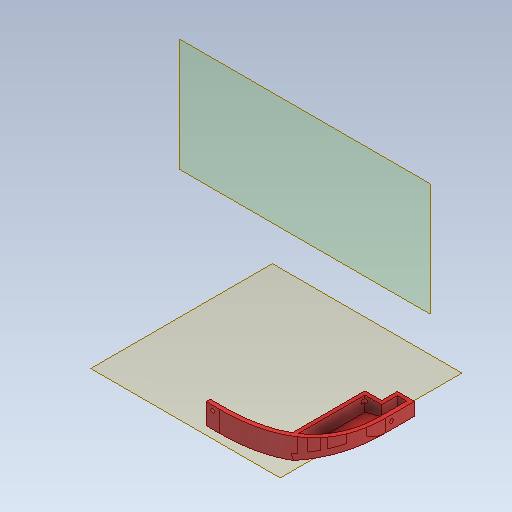
# Autodesk Inventor part: canto
Saved by Autodesk Inventor 2020 (Build 240168000, 168)
## iProperties
Created: 2020-04-24
Part Number: canto
Material: Genérico
Document SubType Name: Modeling
Designer: gi-se
Density: 1 g/cm^3
Appearance: Vermelho alaranjado
Author: gi-se
Autodesk Inventor part; units mm, degrees
ref_plane "YZ Plane" through (0, 0, 0) normal (1, 0, 0) x (0, 1, 0)
ref_plane "XZ Plane" through (0, 0, 0) normal (0, 1, 0) x (-1, 0, 0)
ref_plane "XY Plane" through (0, 0, 0) normal (0, 0, 1) x (1, 0, 0)
ref_plane "Plano de trabalho1" through (4.85, -66.1, 3.317814) normal (0, 1, 0) x (-1, 0, 0)
sketch "Esboço7" plane through (4.85, -66.1, 3.317814) normal (0, 1, 0) x (-1, 0, 0)
  spline S0 degree 4 poles (-63.15, 3.682186) (-63.142335, 9.732075) (-62.18363, 17.577122) (-58.839618, 26.416885) (-51.359365, 34.601206) (-41.420425, 41.161438) (-30.747731, 43.972695) (-21.220771, 44.813565) (-13.75, 44.817814) knots 0 0 0 0 0 0.30669719 0.4235016 0.54102531 0.66311948 1 1 1 1 1
  line L0 (0.45, -30.926645) -> (0.45, -16.417814)
  line L1 (14.341169, -44.817814) -> (0.45, -30.926645)
  line L2 (46.75, -44.817814) -> (14.341169, -44.817814)
  line L3 (46.75, 25.38432) -> (46.75, -44.817814)
  line L4 (-9.75, 35.346795) -> (46.75, 25.38432)
  line L5 (-6.75, 44.817814) -> (-6.75, 38.346795)
  line L6 (-13.75, 44.817814) -> (-6.75, 44.817814)
  spline S1 degree 2 poles (-46.75, 37.469642) (-34.671162, 44.817814) (-13.75, 44.817814) knots 0 0 0 1 1 1
  line L7 (-46.75, -44.817814) -> (-46.75, 37.469642)
  line L8 (4.158831, -44.817814) -> (-46.75, -44.817814)
  line L9 (-5.695584, -34.963398) -> (4.158831, -44.817814)
  arc A0 (-6.75, -32.417814) -> (-5.695584, -34.963398) centre (-3.15, -32.417814) ccw
  line L10 (-6.75, -16.417814) -> (-6.75, -32.417814)
  arc A1 (0.45, -16.417814) -> (-6.75, -16.417814) centre (-3.15, -16.417814) ccw
  circle A2 centre (-14.05, -11.017814) radius 0.8
  line L11 (-63.15, 3.682186) -> (-44.75, 3.682186)
  line L12 (-6.75, 42.567814) -> (-6.75, 44.817814)
  line L13 (-6.75, 44.817814) -> (-13.75, 44.817814)
  line L14 (-60.858893, 5.932186) -> (-44.75, 5.932186)
  line L15 (-9, 42.567814) -> (-13.75, 42.567814)
  line L16 (-44.75, 41.3031) -> (-44.75, 2)
  line L17 (-9, 42.567814) -> (-6.75, 42.567814)
  line L18 (-6.75, 44.817814) -> (-6.75, 42.567814)
  line L19 (-6.75, 42.567814) -> (-9.75, 42.567814)
  line L20 (-9.75, 42.567814) -> (-9.75, 44.817814)
  line L21 (-9.75, 44.817814) -> (-6.75, 44.817814)
  line L22 (-9.75, 38.346795) -> (-9.75, 35.346795)
  line L23 (-6.75, 38.346795) -> (-9.75, 38.346795)
  spline S2 degree 5 poles (-13.748721, 42.567814) (-17.011521, 42.565862) (-20.274495, 42.452633) (-23.531674, 42.205009) (-29.595553, 41.442064) (-35.526192, 39.976484) (-38.23954, 39.119482) (-43.237503, 37.094016) (-47.789537, 34.213647) (-49.802218, 32.646807) (-53.452771, 29.089024) (-56.245096, 24.82436) (-57.399397, 22.545019) (-59.2024, 17.936427) (-60.232691, 13.096486) (-60.5712, 10.718215) (-60.773011, 8.327267) (-60.858895, 5.932186) knots 0 0 0 0 0 0 0.24056469 0.24056469 0.24056469 0.44973286 0.44973286 0.44973286 0.6363542 0.6363542 0.6363542 0.82330304 0.82330304 0.82330304 1 1 1 1 1 1
  point P0 (4.85, -3.317814)
  point P1 (-62.348789, 13.492523)
  point P2 (-60.046821, 21.718124)
  point P3 (-56.342657, 28.55399)
  point P4 (-51.235855, 34.164448)
  point P5 (-44.620354, 38.639423)
  point P6 (-36.311689, 41.974216)
  point P7 (-26.092384, 44.080443)
  point P8 (-46.75, 5.932186)
  point P9 (-46.75, 34.756638)
  point P10 (-44.75, 35.999842)
  point P11 (-13.749358, 42.567814)
  point P12 (-46.75, 3.682186)
  dimension "d24" = 2
  dimension "d37" = 3
  constraints: 22 end point, 6 perpendicular, 4 parallel, 2 point on line, 13 other
  measures "d24" distance between parallel lines of L7 L16
  measures "d37" distance of L12.start L19.end
sketch "Esboço7 outline for Extrusão6" plane through (4.85, -66.1, 3.317814) normal (0, 1, 0) x (-1, 0, 0)
  line L0 (-44.75, 3.682186) -> (-44.750011, 35.999861)
  spline S0 degree 5 poles (-13.748721, 42.567814) (-17.011521, 42.565862) (-20.274495, 42.452633) (-23.531674, 42.205009) (-29.595553, 41.442064) (-35.526192, 39.976484) (-38.23954, 39.119482) (-41.167958, 37.932717) (-43.943286, 36.452458) (-44.213822, 36.304492) (-44.482758, 36.153642) (-44.750023, 35.999881) knots 0 0 0 0 0 0 0.50916763 0.50916763 0.50916763 0.95188291 0.95188291 0.95188291 1 1 1 1 1 1
  line L1 (-13.748721, 42.567814) -> (-9.75, 42.567814)
  line L2 (-9.75, 42.567814) -> (-9.75, 44.817814)
  line L3 (-9.75, 44.817814) -> (-13.75, 44.817814)
  spline S1 degree 4 poles (-63.15, 3.682186) (-63.142335, 9.732075) (-62.18363, 17.577122) (-58.839618, 26.416885) (-51.359365, 34.601206) (-41.420425, 41.161438) (-30.747731, 43.972695) (-21.220771, 44.813565) (-13.75, 44.817814) knots 0 0 0 0 0 0.30669719 0.4235016 0.54102531 0.66311948 1 1 1 1 1
  line L4 (-63.15, 3.682186) -> (-44.75, 3.682186)
  line L5 (-46.75, 5.932186) -> (-60.858895, 5.932186)
  spline S2 degree 5 poles (-46.749999, 34.756636) (-48.204588, 33.780364) (-49.594289, 32.707372) (-50.905012, 31.535519) (-53.882304, 28.433006) (-56.245096, 24.82436) (-57.399397, 22.545019) (-59.2024, 17.936427) (-60.232691, 13.096486) (-60.5712, 10.718215) (-60.773011, 8.327267) (-60.858895, 5.932186) knots 0 0 0 0 0 0 0.26208571 0.26208571 0.26208571 0.64144447 0.64144447 0.64144447 1 1 1 1 1 1
  line L6 (-46.75, 34.756638) -> (-46.75, 5.932186)
extrude "Extrusão6" add sketch "Esboço7 outline for Extrusão6" along normal blind 11.3
sketch "Esboço8" plane through (68, -66.1, 7) normal (0, 0, -1) x (-1, 0, 0)
  line L0 (16.4, 0) -> (16.4, 11.3) projected
  line L1 (16.4, 0) -> (0, 4.3)
  line L2 (0, 4.3) -> (-5, 0)
  line L3 (-5, 0) -> (12, -6)
  line L4 (12, -6) -> (16.4, 0)
  point P0 (68, 66.1)
  constraints: 8 end point, 1 other
sketch "Esboço8 outline for Extrusão7" plane through (68, -66.1, 7) normal (0, 0, -1) x (-1, 0, 0)
  line L0 (0, 4.3) -> (-5, 0)
  line L1 (16.4, 0) -> (0, 4.3)
  line L2 (12, -6) -> (16.4, 0)
  line L3 (-5, 0) -> (12, -6)
extrude "Extrusão7" cut sketch "Esboço8 outline for Extrusão7" against normal blind 48.25
sketch "Esboço9" plane through (68, -54.8, 7) normal (0, 0, -1) x (-1, 0, 0)
  line L0 (16.4, -11.3) -> (2.291107, -7.600717)
  line L1 (0, -7) -> (0, 0)
  line L2 (16.4, -11.3) -> (0, -7)
  line L3 (0, -7) -> (0.800313, -3.947643)
  line L4 (0.800313, -3.947643) -> (17.200313, -8.247643)
  line L5 (17.200313, -8.247643) -> (16.4, -11.3)
  point P0 (68, 54.8)
  constraints: 8 end point, 2 parallel, 1 perpendicular
sketch "Esboço9 outline for Extrusão8" plane through (68, -54.8, 7) normal (0, 0, -1) x (-1, 0, 0)
  line L0 (16.4, -11.3) -> (17.200313, -8.247643)
  line L1 (2.291107, -7.600717) -> (16.4, -11.3)
  line L2 (0, -7) -> (2.291107, -7.600717)
  line L3 (0.800313, -3.947643) -> (0, -7)
  line L4 (17.200313, -8.247643) -> (0.800313, -3.947643)
extrude "Extrusão8" add sketch "Esboço9 outline for Extrusão8" against normal blind 48
sketch "Esboço10" plane through (4.85, -54.8, 3.317814) normal (0, 1, 0) x (1, 0, 0)
  spline S0 degree 2 poles (63.15, -3.682186) (63.15, -44.817814) (13.75, -44.817814) knots 1 1 1 2 2 2
  line L0 (63.15, -3.682186) -> (46.75, -3.682186)
  line L1 (63.15, -3.682186) -> (63.15, -51.682186)
  line L2 (63.15, -51.682186) -> (45.949687, -51.682186)
  line L3 (45.949687, -51.682186) -> (45.949687, -3.682186)
  line L4 (45.949687, -3.682186) -> (63.15, -3.682186)
  point P0 (-4.85, 3.317814)
  point P1 (45.949687, -37.905329)
  constraints: 8 end point, 2 parallel, 1 perpendicular, 1 vertical
sketch "Esboço10 outline for Extrusão9" plane through (4.85, -54.8, 3.317814) normal (0, 1, 0) x (1, 0, 0)
  line L0 (45.949687, -51.682186) -> (63.15, -51.682186)
  line L1 (45.949687, -37.905329) -> (45.949687, -51.682186)
  spline S0 degree 2 poles (63.15, -3.682186) (63.15, -27.955151) (45.949687, -37.905329) knots 0 0 0 1 1 1
  line L2 (63.15, -51.682186) -> (63.15, -3.682186)
extrude "Extrusão9" cut sketch "Esboço10 outline for Extrusão9" against normal blind 48
sketch "Esboço11" plane through (68, -54.8, 7) normal (0, 0, -1) x (-1, 0, 0)
  line L0 (16.4, -11.3) -> (18.4, -11.3) projected
  line L1 (18.4, -11.3) -> (18.4, 0) projected
  line L2 (0, 0) -> (18.4, 0) projected
  line L3 (0, -7) -> (0, 0) projected
  line L4 (0, -7) -> (16.4, -11.3) projected
  line L5 (16.4, -11.3) -> (0, 14.8) projected
  point P0 (68, 54.8)
  point P1 (9.299617, 0)
sketch "Esboço11 outline for Extrusão10" plane through (68, -54.8, 7) normal (0, 0, -1) x (-1, 0, 0)
  line L0 (0, 0) -> (0, -7)
  line L1 (9.299617, 0) -> (0, 0)
  line L2 (16.4, -11.3) -> (9.299617, 0)
  line L3 (0, -7) -> (16.4, -11.3)
extrude "Extrusão10" add sketch "Esboço11 outline for Extrusão10" along normal blind 15.5
sketch "Esboço12" plane through (49.6, -66.1, 7) normal (0, 0, -1) x (-1, 0, 0)
  line L0 (91.5, 0) -> (-2, 0)
  line L1 (117.6, 26.1) -> (91.5, 0)
  line L2 (117.6, 50.1) -> (117.6, 26.1)
  line L3 (93.6, 50.1) -> (117.6, 50.1)
  line L4 (93.6, 82.1) -> (93.6, 50.1)
  line L5 (117.6, 82.1) -> (93.6, 82.1)
  line L6 (117.6, 106.1) -> (117.6, 82.1)
  line L7 (91.5, 132.2) -> (117.6, 106.1)
  line L8 (-2, 132.2) -> (91.5, 132.2)
  line L9 (-18.4, 106.1) -> (-2, 132.2)
  line L10 (-18.4, 26.1) -> (-18.4, 106.1)
  line L11 (-2, 0) -> (-18.4, 26.1)
  spline S0 degree 3 poles (-7.815486, 104.038144) (-7.816082, 104.037708) (-7.816681, 104.03727) (-7.846099, 104.015744) (-7.882015, 103.988404) (-7.95841, 103.925869) (-7.998834, 103.890604) (-8.072489, 103.822008) (-8.110537, 103.784191) (-8.178341, 103.712432) (-8.208164, 103.678549) (-8.253706, 103.624789) (-8.272728, 103.601104) (-8.285509, 103.584876) knots 0 0 0 0 0.00416713 0.00416713 0.20441217 0.20441217 0.40465722 0.40465722 0.60490226 0.60490226 0.8051473 0.8051473 1 1 1 1
  arc A0 (-8.285509, 103.584876) -> (-7.815486, 104.038144) centre (-6.4, 102.1) ccw
  spline S1 degree 3 poles (-7.84364, 32.017255) (-7.866833, 31.999781) (-7.892941, 31.97946) (-7.95841, 31.925869) (-7.998834, 31.890604) (-8.072489, 31.822008) (-8.110537, 31.784191) (-8.168644, 31.722696) (-8.190769, 31.698097) (-8.209846, 31.676205) knots 0 0 0 0 0.20827667 0.20827667 0.5 0.5 0.79172333 0.79172333 1 1 1 1
  arc A1 (-8.209846, 31.676205) -> (-7.84364, 32.017255) centre (-6.4, 30.1) ccw
  line L12 (-2, 11.3) -> (-16.108893, 11.3)
  line L13 (-9.054446, 11.3) -> (0, 11.3)
  line L14 (0, 11.3) -> (0, 0)
  point P0 (49.6, 66.1)
  point P1 (-9.100383, 11.3)
  constraints: 4 end point, 1 horizontal, 1 midpoint, 1 perpendicular, 1 point on line
sketch "Esboço12 outline for Extrusão11" plane through (49.6, -66.1, 7) normal (0, 0, -1) x (-1, 0, 0)
  line L0 (0, 0) -> (0, 11.3)
  line L1 (-2, 0) -> (0, 0)
  line L2 (-9.100383, 11.3) -> (-2, 0)
  line L3 (-2, 11.3) -> (-9.100383, 11.3)
  line L4 (0, 11.3) -> (-2, 11.3)
extrude "Extrusão11" add sketch "Esboço12 outline for Extrusão11" along normal blind 7
sketch "Esboço13" plane through (4.85, -54.8, 3.317814) normal (0, 1, 0) x (1, 0, 0)
  line L0 (46.75, -34.756638) -> (46.75, -5.932186)
  line L1 (46.75, -5.932186) -> (60.858893, -5.932186)
  line L2 (60.858893, -5.932186) -> (60.858893, 1.317814)
  line L3 (55.850383, 1.317814) -> (46.75, 1.317814)
  line L4 (46.75, 1.317814) -> (46.75, -5.932186)
  line L5 (63.15, -3.682186) -> (63.15, 11.817814)
  line L6 (44.75, 3.317814) -> (53.850383, 3.317814)
  line L7 (60.858893, 1.305176) -> (60.858893, 9.817814)
  line L8 (60.858893, 9.817814) -> (55.850383, 9.817814)
  line L9 (55.850383, 9.817814) -> (55.850383, 1.317814)
  line L10 (53.850383, 3.317814) -> (53.850383, 11.817814)
  line L11 (53.850383, 11.817814) -> (63.15, 11.817814)
  line L12 (63.15, -3.682186) -> (63.15, 11.817814)
  line L13 (53.850383, 11.817814) -> (63.15, 11.817814)
  line L14 (53.850383, 3.317814) -> (53.850383, 11.817814)
  line L15 (44.75, 3.317814) -> (53.850383, 3.317814)
  line L16 (44.75, -35.999842) -> (44.75, 3.317814)
  line L17 (13.748721, -42.567814) -> (9.75, -42.567814)
  line L18 (9.75, -42.567814) -> (9.75, -44.817814)
  line L19 (9.75, -44.817814) -> (13.75, -44.817814)
  line L20 (46.75, -5.932186) -> (60.858893, -5.932186)
  line L21 (46.75, -34.756638) -> (46.75, -5.932186)
  point P0 (-4.85, 3.317814)
  point P1 (60.858893, 1.317814)
  dimension "d39" = 2
  dimension "d40" = 2
  dimension "d41" = 2
  dimension "d42" = 0
  dimension "d43" = 0
  constraints: 14 end point, 3 parallel, 1 horizontal, 1 perpendicular, 9 other
  measures "d39" distance between parallel lines of L3 L6
  measures "d40" distance between parallel lines of L10 L9
  measures "d41" distance between parallel lines of L8 L11
  measures "d42" distance from line of L20.end L2
  measures "d43" distance between parallel lines of L7 L2
sketch "Esboço13 outline for Extrusão12" plane through (4.85, -54.8, 3.317814) normal (0, 1, 0) x (1, 0, 0)
  line L0 (46.75, 1.317814) -> (46.75, -5.932186)
  line L1 (55.850383, 1.317814) -> (46.75, 1.317814)
  line L2 (55.850383, 9.817814) -> (55.850383, 1.317814)
  line L3 (60.858893, 9.817814) -> (55.850383, 9.817814)
  line L4 (60.858893, 1.317814) -> (60.858893, 9.817814)
  line L5 (60.858893, -5.932186) -> (60.858893, 1.317814)
  line L6 (46.75, -5.932186) -> (60.858893, -5.932186)
extrude "Extrusão12" cut sketch "Esboço13 outline for Extrusão12" against normal blind 12.25
sketch "Esboço14" plane through (65.708893, -62.400717, 9.25) normal (0, 0, -1) x (-1, 0, 0)
  line L0 (14.108893, -0.437088) -> (0, 3.262195)
  line L1 (0, 3.262195) -> (0, 0)
  line L2 (14.108893, -3.699283) -> (0, 0)
  line L3 (14.108893, -0.437088) -> (14.108893, -3.699283)
  point P0 (65.708893, 62.400717)
sketch "Esboço14 outline for Extrusão13" plane through (65.708893, -62.400717, 9.25) normal (0, 0, -1) x (-1, 0, 0)
  line L0 (0, 3.262195) -> (0, 0)
  line L1 (14.108893, -0.437088) -> (0, 3.262195)
  line L2 (14.108893, -3.699283) -> (14.108893, -0.437088)
  line L3 (0, 0) -> (14.108893, -3.699283)
extrude "Extrusão13" add sketch "Esboço14 outline for Extrusão13" along normal blind 17.25
sketch "Esboço15" plane through (4.85, -66.1, 3.317814) normal (0, -1, 0) x (1, 0, 0)
  line L0 (9.75, 42.567814) -> (9.75, 44.817814)
  line L1 (9.75, 42.567814) -> (16.75, 42.567814)
  line L2 (16.75, 42.567814) -> (21.75, 42.567814)
  line L3 (21.75, 42.567814) -> (21.75, 38.067814)
  line L4 (16.75, 38.067814) -> (16.75, 42.567814)
  circle A0 centre (19.25, 38.067814) radius 1
  arc A1 (16.75, 38.067814) -> (21.75, 38.067814) centre (19.25, 38.067814) ccw
  line L5 (44.75, 3.682186) -> (44.75, -1.317814)
  line L6 (44.75, -1.317814) -> (40.25, -1.317814)
  line L7 (40.25, 3.682186) -> (44.75, 3.682186)
  circle A2 centre (40.25, 1.182186) radius 1
  arc A3 (40.25, 3.682186) -> (40.25, -1.317814) centre (40.25, 1.182186) ccw
  line L8 (60.858893, -9.817814) -> (60.858893, 5.932186)
  line L9 (46.75, 34.756638) -> (46.75, -1.317814)
  line L10 (46.75, -1.317814) -> (55.850383, -1.317814)
  line L11 (55.850383, -1.317814) -> (55.850383, -9.817814)
  line L12 (55.850383, -9.817814) -> (60.858893, -9.817814)
  line L13 (63.15, 3.682186) -> (63.15, -11.817814)
  line L14 (53.850383, -11.817814) -> (63.15, -11.817814)
  line L15 (53.850383, -3.317814) -> (53.850383, -11.817814)
  line L16 (44.75, -3.317814) -> (53.850383, -3.317814)
  line L17 (44.75, 35.999842) -> (44.75, -3.317814)
  spline S0 degree 5 poles (44.750023, 35.999881) (44.482758, 36.153642) (44.213822, 36.304492) (43.943286, 36.452458) (41.167958, 37.932717) (38.23954, 39.119482) (35.526192, 39.976484) (29.595553, 41.442064) (23.531674, 42.205009) (20.274495, 42.452633) (17.011521, 42.565862) (13.748721, 42.567814) knots 0 0 0 0 0 0 0.04811709 0.04811709 0.04811709 0.49083237 0.49083237 0.49083237 1 1 1 1 1 1
  line L18 (13.748721, 42.567814) -> (9.75, 42.567814)
  line L19 (9.75, 42.567814) -> (9.75, 44.817814)
  line L20 (9.75, 44.817814) -> (13.75, 44.817814)
  point P0 (-4.85, -3.317814)
  point P1 (21.75, 42.266312)
  point P2 (16.75, 42.526888)
  dimension "d52" = 2
  dimension "d54" = 2
  dimension "d55" = 7
  dimension "d56" = 1.5
  dimension "d58" = 0
  constraints: 14 end point, 4 centre point, 4 point on circle, 2 coincident, 2 horizontal, 2 parallel, 2 perpendicular, 9 other
  measures "d52" diameter of A0
  measures "d54" diameter of A2
  measures "d56" radial gap between concentric circles of A3 A2
  measures "d58" distance between parallel lines of L10 L6
sketch "Esboço15 outline for Extrusão14" plane through (4.85, -66.1, 3.317814) normal (0, -1, 0) x (1, 0, 0)
  arc A0 (16.75, 38.067814) -> (21.75, 38.067814) centre (19.25, 38.067814) ccw
  line L0 (16.75, 42.526888) -> (16.75, 38.067814)
  line L1 (21.75, 38.067814) -> (21.75, 42.266312)
  spline S0 degree 5 poles (21.749999, 42.266301) (20.75162, 42.344864) (19.752138, 42.409407) (18.751883, 42.460762) (17.751102, 42.499686) (16.75, 42.526889) knots 0 0 0 0 0 0 1 1 1 1 1 1
  circle A1 centre (19.25, 38.067814) radius 1
  arc A2 (40.25, 3.682186) -> (40.25, -1.317814) centre (40.25, 1.182186) ccw
  line L2 (44.75, 3.682186) -> (40.25, 3.682186)
  line L3 (40.25, -1.317814) -> (44.75, -1.317814)
  line L4 (44.75, -1.317814) -> (44.75, 3.682186)
  circle A3 centre (40.25, 1.182186) radius 1
extrude "Extrusão14" add sketch "Esboço15 outline for Extrusão14" against normal blind 2
sketch "Esboço16" plane through (58.700383, -54.8, -8.5) normal (-0.8467201, 0.5320387, 0) x (0, 0, 1)
  line L0 (8.5, -8.732927) -> (8.5, 0)
  line L1 (8.5, -7.235594) -> (0, -7.235594)
  line L2 (0, -7.235594) -> (0, -16)
  line L3 (0, -16) -> (8.5, -16)
  line L4 (8.5, -16) -> (8.5, -7.235594)
  point P0 (8.5, 15.169386)
  point P1 (8.5, -8.732927)
  constraints: 8 end point, 2 parallel, 1 horizontal, 1 perpendicular, 1 point on line
sketch "Esboço16 outline for Extrusão15" plane through (58.700383, -54.8, -8.5) normal (-0.8467201, 0.5320387, 0) x (0, 0, 1)
  line L0 (0, -16) -> (8.5, -16)
  line L1 (0, -7.235594) -> (0, -16)
  line L2 (8.5, -7.235594) -> (0, -7.235594)
  line L3 (8.5, -8.732927) -> (8.5, -7.235594)
  line L4 (8.5, -16) -> (8.5, -8.732927)
extrude "Extrusão15" cut sketch "Esboço16 outline for Extrusão15" along normal blind 2
sketch "Esboço17" plane through (4.85, -54.8, 3.317814) normal (0, 1, 0) x (1, 0, 0)
  line L0 (9.75, -44.817814) -> (13.75, -44.817814)
  line L1 (9.75, -44.817814) -> (13.75, -44.817814)
  line L2 (13.75, -44.817814) -> (6.75, -44.817814)
  line L3 (6.75, -44.817814) -> (6.75, -42.567814)
  line L4 (6.75, -42.567814) -> (13.75, -42.567814)
  line L5 (13.75, -42.567814) -> (13.75, -44.817814)
  point P0 (-4.85, 3.317814)
  dimension "d63" = 7
  constraints: 8 end point, 2 parallel, 1 horizontal, 1 perpendicular
  measures "d63" distance of L3.end L4.end
sketch "Esboço17 outline for Extrusão16" plane through (4.85, -54.8, 3.317814) normal (0, 1, 0) x (1, 0, 0)
  line L0 (13.75, -44.817814) -> (13.75, -42.567814)
  line L1 (9.75, -44.817814) -> (13.75, -44.817814)
  line L2 (6.75, -44.817814) -> (9.75, -44.817814)
  line L3 (6.75, -42.567814) -> (6.75, -44.817814)
  line L4 (13.75, -42.567814) -> (6.75, -42.567814)
extrude "Extrusão16" add sketch "Esboço17 outline for Extrusão16" against normal blind 11.3
sketch "Esboço18" plane through (18.6, -66.1, 48.135628) normal (0, 0, 1) x (1, 0, 0)
  circle A0 centre (-3.5, 8.8) radius 1
  line L0 (-7, 11.3) -> (0, 11.3) projected
  line L1 (-7, 11.3) -> (-7, 0) projected
  point P0 (-18.6, 66.1)
  dimension "d66" = 2
  dimension "d67" = 2.5
  dimension "d68" = 3.5
  constraints: 1 centre point
  measures "d66" diameter of A0
  measures "d67" distance from line of L0 A0.centre
  measures "d68" distance from line of L1 A0.centre
sketch "Esboço18 outline for Extrusão18" plane through (18.6, -66.1, 48.135628) normal (0, 0, 1) x (1, 0, 0)
  circle A0 centre (-3.5, 8.8) radius 1
extrude "Extrusão18" cut sketch "Esboço18 outline for Extrusão18" against normal blind 4.25
sketch "Esboço20" plane through (49.6, -66.1, 0) normal (0, 0, -1) x (-1, 0, 0)
  circle A0 centre (-2.5, 8.8) radius 1
  line L0 (0, 0) -> (0, 11.3)
  line L1 (0, 11.3) -> (-9.100383, 11.3)
  point P0 (49.6, 66.1)
  dimension "d77" = 2
  dimension "d78" = 2.5
  dimension "d79" = 2.5
  constraints: 1 centre point
  measures "d77" diameter of A0
  measures "d78" distance from line of L0 A0.centre
  measures "d79" distance from line of L1 A0.centre
sketch "Esboço20 outline for Extrusão19" plane through (49.6, -66.1, 0) normal (0, 0, -1) x (-1, 0, 0)
  circle A0 centre (-2.5, 8.8) radius 1
extrude "Extrusão19" cut sketch "Esboço20 outline for Extrusão19" against normal blind 4
ref_plane "Plano de trabalho2" through (-12.38612, -3.378396, -29.474354) normal (0, 0, -1) x (-1, 0, 0)
sketch "Esboço21" plane through (68, -61.8, 7) normal (1, 0, 0) x (0, 0, -1)
  line L0 (7, -4.3) -> (7, 7) projected
  circle A0 centre (3, 4) radius 1
  line L1 (0, 7) -> (15.5, 7) projected
  line L2 (0, 0) -> (0, 7) projected
  point P0 (7, 61.8)
  dimension "d82" = 2
  dimension "d83" = 3
  dimension "d84" = 3
  constraints: 1 centre point
  measures "d82" diameter of A0
  measures "d83" distance from line of L1 A0.centre
  measures "d84" distance from line of L2 A0.centre
sketch "Esboço21 outline for Extrusão20" plane through (68, -61.8, 7) normal (1, 0, 0) x (0, 0, -1)
  circle A0 centre (3, 4) radius 1
extrude "Extrusão20" cut sketch "Esboço21 outline for Extrusão20" against normal blind 4
